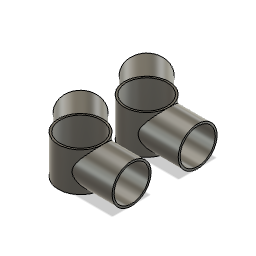
hindge2 (Autodesk Fusion 360 design; units mm, degrees)
Autodesk Fusion 360 part; units mm, degrees
sketch "Sketch1" plane through (0, 0, 0) normal (0, 1, 0) x (1, 0, 0)
  circle A0 centre (0, 0) radius 21.5
  circle A1 centre (0, 0) radius 23.5
  circle A2 centre (0, 0) radius 2
  dimension "d1" = 43
  dimension "d2" = 47
  dimension "d3" = 4
  constraint coincident A0.centre A1.centre
  constraint concentric A1 A2
  measures "d1" diameter of A0
  measures "d2" diameter of A1
  measures "d3" diameter of A2
extrude "Extrude1" add sketch "Sketch1" along normal blind 3 contours A0 in component "Component"
sketch "Sketch2" plane through (0, 0, 0) normal (0, -1, 0) x (1, 0, 0)
  circle A0 centre (0, 0) radius 2
  circle A1 centre (0, 0) radius 21.5
  circle A2 centre (0, 0) radius 21.5
  circle A3 centre (0, 0) radius 23.5
  dimension "d6" = 47
  constraint coincident A0.centre A1.centre
  constraint concentric A2 A3
  measures "d6" diameter of A3
extrude "Extrude2" add sketch "Sketch2" against normal blind 41 contours A3 in component "Component"
ref_plane "WorkPlane1" through (0, 20.5, 0) normal (0, 1, 0) x (-1, 0, 0)
sketch "Sketch3" plane through (0, 20.5, 0) normal (0, 1, 0) x (1, 0, 0)
  line L0 (0, 0) -> (70, 0)
  line L1 (0, 0) -> (-70.7107, 70.7107)
  line L2 (0, 0) -> (100, 0) construction
  dimension "d9" = 135
  dimension "d10" = 100
  constraint coincident L0.start L1.start
  constraint horizontal L0
  constraint horizontal L2
  measures "d9" angle of L1 L2
  measures "d10" distance of L0.start L1.end
pipe "Pipe1" add diameter 41 wall 2 path "Sketch3" along L1 for 0.535 of its length starting at (0, 20.5, 0) heading (-0.7071, 0, -0.7071) in component "Component"
ref_plane "WorkPlane2" through (0, 20.5, 0) normal (0, 1, 0) x (-1, 0, 0)
sketch "Sketch4" plane through (0, 20.5, 0) normal (0, 1, 0) x (1, 0, 0)
  line L0 (0, 0) -> (100, 0)
  constraint coincident L0.start origin
  constraint horizontal L0
pipe "Pipe2" add diameter 41 wall 2 path "Sketch4" along L0 for 0.539 of its length starting at (0, 20.5, 0) heading (1, 0, 0) in component "Component"
hole "Hole1" at (0, 41, 0) direction (0, -1, 0) diameter 43 depth 38 tip angle 118 in component "Component"
extrude "Extrude3" add 1 faces at (21.0689, 0, -1.5606) along direction (0, 1, 0) blind 3 in component "Component"
sketch "Sketch5" plane through (0, 3, 0) normal (0, 1, 0) x (-1, 0, 0)
  circle A0 centre (0, 0) radius 16.5072
  circle A1 centre (0, 0) radius 21.5
  circle A2 centre (0, 0) radius 2
  dimension "d24" = 4
  constraint coincident A0.centre A1.centre
  measures "d24" diameter of A2
extrude "Extrude4" add sketch "Sketch5" against normal blind 3 contours A0 in component "Component"
component "Component" placed x (1, 0, 0) y (0, 1, 0) z (0, 0, 1) at (0, 0, 0)
component "Component" placed x (1, 0, 0) y (0, 1, 0) z (0, 0, 1) at (-0.8456, 0, 68.9856)
